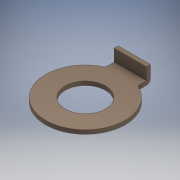
# Autodesk Inventor part: podkładka z jednym uchem
Saved by Autodesk Inventor 2017 SP1 (Build 210196100, 196)
## iProperties
Created: 2021-02-08
Part Number: podkładka z jednym uchem
Material: Stal
Document SubType Name: Modeling
Designer: Napoleon
Mass: 0.264158 g
Surface Area: 1.60802 cm^2
Volume: 0.0336507 cm^3
Density: 7.85 g/cm^3
Appearance: Anodowana - ciemnobrązowa
Author: Napoleon
Autodesk Inventor part; units mm, degrees
ref_plane "YZ Plane" through (0, 0, 0) normal (1, 0, 0) x (0, 1, 0)
ref_plane "XZ Plane" through (0, 0, 0) normal (0, 1, 0) x (-1, 0, 0)
ref_plane "XY Plane" through (0, 0, 0) normal (0, 0, 1) x (1, 0, 0)
sketch "Szkic1" plane through (0, 0, 0) normal (0, 0, 1) x (1, 0, 0)
  circle A0 centre (0, 0) radius 2.5
  arc A1 (-2.1413, 4.4351) -> (2.1413, 4.4351) centre (0, 0) ccw
  line L0 (-2, 6.075) -> (2, 6.075)
  line L1 (-2, 6.075) -> (-2, 4.6603)
  line L2 (2, 6.075) -> (2, 4.6603)
  arc A2 (-2.1413, 4.4351) -> (-2, 4.6603) centre (-2.25, 4.6603) ccw
  arc A3 (2, 4.6603) -> (2.1413, 4.4351) centre (2.25, 4.6603) ccw
  point P0 (-2, 4.5006)
  point P1 (2, 4.5006)
  dimension "d0" = 5
  dimension "d1" = 9.85
  dimension "d3" = 4
  dimension "d4" = 0.25
  constraints: 8 point on circle, 6 end point, 4 centre point, 4 tangent, 2 coincident, 2 point on line, 2 vertical, 1 equal radius, 1 horizontal
  measures "d0" diameter of A0
  measures "d1" diameter of A1
  measures "d3" distance of L0.start L0.end
  measures "d4" radius of A2
extrude "Wyciągnięcie proste1" add sketch "Szkic1" along normal mid plane 0.5
sketch "Szkic2" plane through (0, 0, 0.25) normal (0, 0, 1) x (1, 0, 0)
  line L0 (2, 6.075) -> (-2, 6.075) projected
  line L1 (-2, 6.075) -> (2, 6.075)
  line L2 (2, 6.075) -> (2, 5.575)
  line L3 (2, 5.575) -> (-2, 5.575)
  line L4 (-2, 5.575) -> (-2, 6.075)
  dimension "d7" = 0.5
  constraints: 8 end point, 2 parallel, 1 horizontal, 1 perpendicular
  measures "d7" distance of L1.end L2.end
extrude "Wyciągnięcie proste2" add sketch "Szkic2" along normal blind 1.5
fillet "Zaokrąglenie1" radius 0.5 1 edges at (0, 6.075, -0.25)
